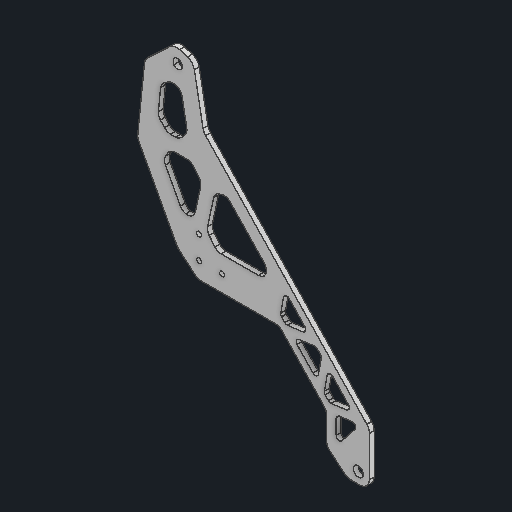
# Autodesk Inventor part: ShoulderBracketRedesign
Saved by Autodesk Inventor 2025.2 (Build 292293000, 293)
## iProperties
Created: 2025-01-19
Part Number: ShoulderBracketRedesign
Material: Generic
Document SubType Name: Sheet Metal
Designer: valer
Density: 1 g/cm^3
Sheet Metal Rule: Default
Appearance: Default
Author: valer
Autodesk Inventor part; units mm, degrees
ref_plane "YZ Plane" through (0, 0, 0) normal (1, 0, 0) x (0, 1, 0)
ref_plane "XZ Plane" through (0, 0, 0) normal (0, 1, 0) x (-1, 0, 0)
ref_plane "XY Plane" through (0, 0, 0) normal (0, 0, 1) x (1, 0, 0)
sketch "Profile" plane through (0, 0, 0) normal (0, 0, 1) x (1, 0, 0)
  circle A0 centre (-41.4125, 89.9251) radius 3.175 construction
  circle A1 centre (-27.9037, 3.7025) radius 1.5875
  circle A2 centre (-27.8803, -10.7935) radius 1.5875
  circle A3 centre (-13.3843, -10.7935) radius 1.5875
  circle A4 centre (72.5232, -75.6183) radius 3.175
  line L0 (65.5232, -82.6183) -> (79.5232, -82.6183)
  line L1 (79.5232, -82.6183) -> (79.5232, -48.9428)
  line L2 (-96.035, 0) -> (108.7829, 0) construction
  line L3 (0, -118.977) -> (0, 135.5337) construction
  line L4 (-36.2503, -15.7274) -> (-46.8807, -15.7402) construction
  line L5 (-41.4125, 89.9251) -> (-41.2847, -15.7335) construction
  line L6 (72.5232, -75.6183) -> (72.5232, 0) construction
  line L7 (72.5232, -75.6183) -> (0, -75.6183) construction
  line L8 (-41.4125, 89.9251) -> (0, 89.9251) construction
  line L9 (52.5232, -52.4886) -> (52.5232, -71.7101)
  line L10 (52.5232, -71.7101) -> (65.5232, -82.6183)
  line L11 (58.5232, -51.7007) -> (58.5232, -68.7101)
  line L12 (58.5232, -68.7101) -> (73.5232, -49.7307)
  line L13 (73.5232, -49.7307) -> (58.5232, -51.7007)
  line L14 (-26.3576, -21.2033) -> (22.6626, -21.124)
  line L15 (-12.3805, -21.1807) -> (-26.3576, -21.2033) construction
  arc A5 (-30.4769, -19.6947) -> (-26.3576, -21.2033) centre (-26.3679, -14.8534) ccw
  line L16 (-30.4769, -19.6947) -> (-40.5808, -11.1193)
  spline S0 degree 3 poles (-40.5808, -11.1193) (-41.0993, -10.6401) (-41.5339, -10.0774) (-41.8663, -9.4545) knots 15 15 15 15 16 16 16 16
  line L17 (-41.8663, -9.4545) -> (-65.7822, 35.3495)
  spline S1 degree 3 poles (-65.7822, 35.3495) (-66.3749, 36.46) (-66.6224, 37.7222) (-66.4956, 38.9741) knots 17 17 17 17 18 18 18 18
  line L18 (-66.4956, 38.9741) -> (-62.271, 79.8043)
  spline S2 degree 3 poles (-62.271, 79.8043) (-62.1143, 81.3192) (-61.4154, 82.7265) (-60.3032, 83.7671) knots 19 19 19 19 20 20 20 20
  line L19 (-60.3032, 83.7671) -> (-46.2664, 96.8991)
  spline S3 degree 3 poles (-46.2664, 96.8991) (-44.604, 98.4544) (-42.2333, 98.9949) (-40.061, 98.3138) knots 21 21 21 21 22 22 22 22
  line L20 (-40.061, 98.3138) -> (-35.1427, 96.7719)
  spline S4 degree 3 poles (-35.1427, 96.7719) (-32.9139, 96.0731) (-31.2526, 94.2014) (-30.8232, 91.9054) knots 23 23 23 23 24 24 24 24
  line L21 (-30.8232, 91.9054) -> (-25.3621, 62.7037)
  spline S5 degree 3 poles (-25.3621, 62.7037) (-25.1376, 61.5033) (-24.57, 60.3937) (-23.7279, 59.5092) knots 25 25 25 25 26 26 26 26
  line L22 (-23.7279, 59.5092) -> (22.9055, 10.5268)
  line L23 (-49.8219, 75.3487) -> (-47.1489, 77.1074)
  spline S6 degree 3 poles (-47.1489, 77.1074) (-45.8817, 77.9412) (-44.3069, 78.1616) (-42.8594, 77.7078) knots 12 12 12 12 13 13 13 13
  line L24 (-42.8594, 77.7078) -> (-42.0163, 77.4435)
  spline S7 degree 3 poles (-42.0163, 77.4435) (-40.2333, 76.8844) (-38.9042, 75.3871) (-38.5607, 73.5503) knots 0 0 0 0 1 1 1 1
  line L25 (-38.5607, 73.5503) -> (-35.6113, 57.7788)
  spline S8 degree 3 poles (-35.6113, 57.7788) (-35.3352, 56.3029) (-35.7298, 54.7807) (-36.6881, 53.6247) knots 2 2 2 2 3 3 3 3
  line L26 (-36.6881, 53.6247) -> (-38.8188, 51.0544)
  spline S9 degree 3 poles (-38.8188, 51.0544) (-39.7771, 49.8984) (-41.1997, 49.2284) (-42.7012, 49.226) knots 4 4 4 4 5 5 5 5
  line L27 (-42.7012, 49.226) -> (-45.8259, 49.2209)
  spline S10 degree 3 poles (-45.8259, 49.2209) (-47.2581, 49.2186) (-48.6241, 49.8241) (-49.5841, 50.8869) knots 6 6 6 6 7 7 7 7
  line L28 (-49.5841, 50.8869) -> (-52.2345, 53.8208)
  spline S11 degree 3 poles (-52.2345, 53.8208) (-53.1945, 54.8836) (-53.6585, 56.3038) (-53.5111, 57.7285) knots 8 8 8 8 9 9 9 9
  line L29 (-53.5111, 57.7285) -> (-52.071, 71.6471)
  spline S12 degree 3 poles (-52.071, 71.6471) (-51.9149, 73.156) (-51.0892, 74.5149) (-49.8219, 75.3487) knots 10 10 10 10 11 11 11 11
  line L30 (-43.0804, 40.8028) -> (-35.4056, 40.8152)
  spline S13 degree 3 poles (-47.4082, 38.345) (-46.497, 39.867) (-44.8544, 40.7999) (-43.0804, 40.8028) knots 10 10 10 10 11 11 11 11
  line L31 (-48.9274, 35.8074) -> (-47.4082, 38.345)
  spline S14 degree 3 poles (-49.0496, 30.8319) (-49.885, 32.3969) (-49.8386, 34.2853) (-48.9274, 35.8074) knots 8 8 8 8 9 9 9 9
  line L32 (-39.6374, 13.199) -> (-49.0496, 30.8319)
  spline S15 degree 3 poles (-35.4056, 40.8152) (-33.877, 40.8176) (-32.4294, 40.128) (-31.4681, 38.9395) knots 1 1 1 1 2 2 2 2
  line L33 (-31.4681, 38.9395) -> (-27.8607, 34.4789)
  spline S16 degree 3 poles (-27.8607, 34.4789) (-26.8994, 33.2903) (-26.5278, 31.7305) (-26.8499, 30.2362) knots 3 3 3 3 4 4 4 4
  line L34 (-26.8499, 30.2362) -> (-30.2392, 14.5138)
  spline S17 degree 3 poles (-36.2441, 10.6387) (-37.6966, 10.9518) (-38.9377, 11.8882) (-39.6374, 13.199) knots 6 6 6 6 7 7 7 7
  spline S18 degree 3 poles (-30.2392, 14.5138) (-30.8273, 11.7855) (-33.5158, 10.0505) (-36.2441, 10.6387) knots 5 5 5 5 6 6 6 6
  spline S19 degree 3 poles (-18.6657, 28.2333) (-18.2711, 30.0637) (-16.8968, 31.5259) (-15.0943, 32.0331) knots 1 1 1 1 2 2 2 2
  line L35 (-15.0943, 32.0331) -> (-13.3719, 32.5177)
  spline S20 degree 3 poles (-13.3719, 32.5177) (-11.5694, 33.0248) (-9.6342, 32.4937) (-8.3431, 31.1376) knots 3 3 3 3 4 4 4 4
  line L36 (-8.3431, 31.1376) -> (13.257, 8.4494)
  spline S21 degree 3 poles (13.257, 8.4494) (15.1815, 6.428) (15.1029, 3.2292) (13.0815, 1.3048) knots 5 5 5 5 6 6 6 6
  spline S22 degree 3 poles (13.0815, 1.3048) (12.144, 0.4122) (10.8996, -0.0866) (9.6051, -0.0887) knots 6 6 6 6 7 7 7 7
  line L37 (9.6051, -0.0887) -> (-13.943, -0.1268)
  spline S23 degree 3 poles (-13.943, -0.1268) (-15.4717, -0.1293) (-16.9193, 0.5603) (-17.8806, 1.7489) knots 8 8 8 8 9 9 9 9
  line L38 (-17.8806, 1.7489) -> (-21.488, 6.2095)
  spline S24 degree 3 poles (-21.488, 6.2095) (-22.4493, 7.3981) (-22.8208, 8.9579) (-22.4987, 10.4522) knots 10 10 10 10 11 11 11 11
  line L39 (-22.4987, 10.4522) -> (-18.6657, 28.2333)
  line L40 (22.9055, 10.5268) -> (79.5232, -48.9428)
  line L41 (22.6626, -21.124) -> (52.5232, -52.4886)
  line L42 (52.5232, -52.4886) -> (79.5232, -48.9428) construction
  line L43 (52.5232, -71.7101) -> (79.5232, -71.7101) construction
  line L44 (22.6626, -21.124) -> (38.5964, -5.9544) construction
  arc A6 (-43.8125, 88.1251) -> (-43.8125, 91.7251) centre (-41.4125, 89.9251) ccw
  line L45 (-43.8125, 88.1251) -> (-43.8125, 91.7251)
  point P0 (0, 0)
  point P1 (65.5232, -75.6183)
  dimension "d0" = 7
  dimension "d1" = 7
  dimension "d68" = 20
  dimension "d71" = 8.4204
  dimension "d77" = 6
  dimension "d78" = 6
  dimension "d82" = 3
  dimension "d87" = 130
  dimension "d88" = 14
  dimension "d94" = 22
  measures "d0" distance from line of L1 L6.start
  measures "d1" distance from line of L0 L6.start
  measures "d68" distance between parallel lines of L6 L9
  measures "d71" distance between parallel lines of L22 L36
  measures "d77" distance between parallel lines of L9 L11
  measures "d78" distance from line of L1 L12.end
  measures "d82" distance from line of L43 L11.end
  measures "d87" angle of L9 L10
  measures "d88" distance of L0.start L0.end
  measures "d94" distance between parallel lines of L40 L41
extrude "Plate1" add sketch "Profile" along normal blind 3.048
fillet "OuterFilletsFeature" radius 6 6 edges at (22.6626, -21.124, 1.524) (52.5232, -52.4886, 1.524) (52.5232, -71.7101, 1.524) (65.5232, -82.6183, 1.524) (79.5232, -48.9428, 1.524) (79.5232, -82.6183, 1.524)
sketch "ExtensionCuts" plane through (0, 0, 3.048) normal (0, 0, 1) x (1, 0, 0)
  line L0 (54.392, -47.2003) -> (69.1193, -45.2662)
  line L1 (69.1193, -45.2662) -> (53.5993, -28.9644)
  line L2 (53.5993, -28.9644) -> (50.9444, -43.579)
  line L3 (50.9444, -43.579) -> (54.392, -47.2003)
  line L4 (46.6768, -39.0965) -> (49.3318, -24.482)
  line L5 (49.3318, -24.482) -> (45.8842, -20.8607)
  line L6 (45.8842, -20.8607) -> (31.1569, -22.7948)
  line L7 (31.1569, -22.7948) -> (46.6768, -39.0965)
  line L8 (26.8894, -18.3123) -> (41.6166, -16.3782)
  line L9 (41.6166, -16.3782) -> (26.0967, -0.0765)
  line L10 (26.0967, -0.0765) -> (23.4417, -14.691)
  line L11 (23.4417, -14.691) -> (26.8894, -18.3123)
  line L12 (58.5232, -51.7007) -> (73.5232, -49.7307) projected
  line L13 (50.8687, -50.7509) -> (24.4401, -22.991) projected
  line L14 (-23.7279, 59.5092) -> (77.8687, -47.205) projected
  point P0 (0, 0)
  point P1 (60.2627, -51.4722)
  point P2 (68.6394, -50.3721)
  dimension "d113" = 126.111
  dimension "d114" = 126.111
  dimension "d115" = 5
  dimension "d116" = 5
  dimension "d117" = 5
  dimension "d118" = 5
  dimension "d119" = 53.889
  dimension "d120" = 53.889
  dimension "d121" = 5
  dimension "d122" = 126.111
  dimension "d123" = 126.111
  dimension "d124" = 5
  constraints: 24 end point, 8 parallel, 4 collinear, 2 equal length
  measures "d113" angle of L0 L3
  measures "d114" angle of L2 L3
  measures "d115" distance between parallel lines of L12 L0
  measures "d116" distance between parallel lines of L14 L1
  measures "d117" distance between parallel lines of L13 L3
  measures "d118" distance between parallel lines of L2 L4
  measures "d119" angle of L4 L7
  measures "d120" angle of L6 L7
  measures "d121" distance between parallel lines of L6 L8
  measures "d122" angle of L8 L11
  measures "d123" angle of L11 L10
  measures "d124" distance of L2.end L0.start
extrude "ExtensionCutsFeature" cut sketch "ExtensionCuts" against normal blind 3.048
fillet "InnerFilletsFeature" radius 2 15 edges at (26.0967, -0.0765, 1.524) (23.4417, -14.691, 1.524) (26.8894, -18.3123, 1.524) (41.6166, -16.3782, 1.524) (45.8842, -20.8607, 1.524) (49.3318, -24.482, 1.524) (31.1569, -22.7948, 1.524) (46.6768, -39.0965, 1.524) (54.392, -47.2003, 1.524) (50.9444, -43.579, 1.524) (53.5993, -28.9644, 1.524) (69.1193, -45.2662, 1.524) (58.5232, -51.7007, 1.524) (73.5232, -49.7307, 1.524) (58.5232, -68.7101, 1.524)
equation "\"d1\" = d0"
equation "\"BendRadius\" = Thickness"
equation "\"BendReliefWidth\" = Thickness"
equation "\"BendReliefDepth\" = 0.5 * Thickness"
equation "\"CornerReliefSize\" = 4 * Thickness"
equation "\"MinimumRemnant\" = 2 * Thickness"
equation "\"TransitionRadius\" = BendRadius"
equation "\"JacobiRadiusSize\" = BendRadius"
equation "\"GapSize\" = Thickness"
equation "\"Thickness\" = 3.048"
body "Solid1"
